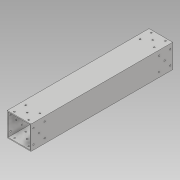
# Autodesk Inventor part: square_tube
Saved by Autodesk Inventor 2017 (Build 210142000, 142)
## iProperties
Part Number: square_tube
Material: Aluminium 6061
Document SubType Name: Modeling
Designer: Max
Mass: 488.16 g
Surface Area: 1817.04 cm^2
Volume: 180.8 cm^3
Density: 2.7 g/cm^3
Appearance: Vorgabe
Author: Max
Autodesk Inventor part; units mm, degrees
ref_plane "YZ Plane" through (0, 0, 0) normal (1, 0, 0) x (0, 1, 0)
ref_plane "XZ Plane" through (0, 0, 0) normal (0, 1, 0) x (-1, 0, 0)
ref_plane "XY Plane" through (0, 0, 0) normal (0, 0, 1) x (1, 0, 0)
sketch "Skizze1" plane through (0, 0, 0) normal (0, 1, 0) x (-1, 0, 0)
  line L0 (-29.25, 29.25) -> (29.25, 29.25)
  line L1 (29.25, 29.25) -> (29.25, -29.25)
  line L2 (29.25, -29.25) -> (-29.25, -29.25)
  line L3 (-29.25, -29.25) -> (-29.25, 29.25)
  line L4 (-29.25, 29.25) -> (29.25, -29.25) construction
  line L5 (29.25, 29.25) -> (-29.25, -29.25) construction
  line L6 (27.25, -27.25) -> (27.25, 27.25)
  line L7 (27.25, 27.25) -> (-27.25, 27.25)
  line L8 (-27.25, 27.25) -> (-27.25, -27.25)
  line L9 (-27.25, -27.25) -> (27.25, -27.25)
  point P0 (0, 0)
  dimension "d0" = 2
  dimension "d1" = 54.5
  dimension "d2" = 54.5
  constraints: 20 end point, 4 parallel, 2 midpoint, 2 perpendicular, 1 horizontal, 3 other
  measures "d0" distance between parallel lines of L6 L1
  measures "d1" distance of L6.start L6.end
  measures "d2" distance of L8.end L6.start
extrude "Extrusion1" add sketch "Skizze1" along normal blind 350
sketch "Skizze2" plane through (-29.25, 0, 29.25) normal (0, 0, 1) x (1, 0, 0)
  line L0 (11.75, 6.25) -> (46.75, 6.25)
  line L1 (46.75, 6.25) -> (46.75, 33.75)
  line L2 (46.75, 33.75) -> (11.75, 33.75)
  line L3 (11.75, 33.75) -> (11.75, 6.25)
  line L4 (11.75, 6.25) -> (46.75, 33.75) construction
  line L5 (46.75, 6.25) -> (11.75, 33.75) construction
  line L6 (58.5, 0) -> (0, 0) projected
  line L7 (58.5, 0) -> (58.5, 350) projected
  line L8 (0, 350) -> (58.5, 350) projected
  line L9 (0, 0) -> (0, 350) projected
  point P0 (29.25, 0)
  point P1 (29.25, 20)
  dimension "d5" = 35
  dimension "d6" = 27.5
  dimension "d7" = 58.5
  dimension "d8" = 29.25
  dimension "d25" = 20
  constraints: 12 end point, 2 midpoint, 2 parallel, 1 horizontal, 1 perpendicular
  measures "d5" distance of L1.end L2.end
  measures "d6" distance of L0.end L1.end
  measures "d7" distance of L6.start L6.end
  measures "d8" distance from line of point (29.25, 20) L9
  measures "d25" distance from line of L6 point (29.25, 20)
hole "Bohrung1" at (0, 20, 29.25) at (-17.5, 6.25, 29.25) at (-17.5, 33.75, 29.25) at (17.5, 6.25, 29.25) at (17.5, 33.75, 29.25) direction (0, 0, -1) diameter 3.4 end up to face face through (-9.0833, 233.3333, 27.25) facing (0, 0, -1) clearance for "Inbusschraube ISO 4762" size "M3" standard "ISO"
mirror "Spiegeln1" about plane through (0, 0, 0) normal (0, 0, 1) of "Bohrung1"
ref_plane "Arbeitsebene2" through (0, 175, 0) normal (0, -1, 0) x (1, 0, 0)
mirror "Spiegeln2" about plane through (0, 175, 0) normal (0, -1, 0) of "Bohrung1", "Spiegeln1"
pattern_circular "Runde Anordnung1" count 2 over 90 about axis through (0, -10, 0) along (0, 1, 0) of "Bohrung1", "Spiegeln1", "Spiegeln2"
ref_plane "Arbeitsebene1" through (0, 0, 0) normal (0, 0, 1) x (1, 0, 0)
ref_plane "Arbeitsebene3" through (0, 350, 0) normal (0, 0, -1) x (1, 0, 0)
ref_plane "Arbeitsebene4" through (0, 350, 0) normal (0, 0, -1) x (1, 0, 0)
ref_plane "Arbeitsebene5" through (0, 0, 0) normal (1, 0, 0) x (0, 0, -1)
ref_plane "Arbeitsebene6" through (0, 0, 0) normal (1, 0, 0) x (0, 0, -1)
ref_plane "Arbeitsebene7" through (0, 350, 0) normal (-1, 0, 0) x (0, 0, -1)
ref_plane "Arbeitsebene8" through (0, 350, 0) normal (-1, 0, 0) x (0, 0, -1)
equation "\"d8\" = 0.5 * d7"
